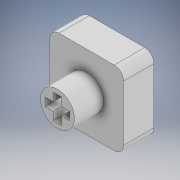
# Autodesk Inventor part: IPC STPT 4 key
Saved by Autodesk Inventor 2022 (Build 260153000, 153)
## iProperties
Created: 2021-12-31
Part Number: IPC STPT 4 key
Material: Generic
Document SubType Name: Modeling
Designer: solor
Density: 1 g/cm^3
Appearance: Default
Author: solor
Autodesk Inventor part; units mm, degrees
ref_plane "YZ Plane" through (0, 0, 0) normal (1, 0, 0) x (0, 1, 0)
ref_plane "XZ Plane" through (0, 0, 0) normal (0, 1, 0) x (-1, 0, 0)
sketch "Sketch1" plane through (0, 0, 0) normal (0, 0, 1) x (1, 0, 0)
  line L0 (14.6962, 12.74) -> (14.6962, 0) construction
  line L1 (10.61, 12.2) -> (1.53, 12.2)
  arc A0 (1.53, 12.2) -> (0, 10.67) centre (1.53, 10.67) ccw
  line L2 (0, 10.67) -> (0, 1.53)
  arc A1 (0, 1.53) -> (1.53, 0) centre (1.53, 1.53) ccw
  line L3 (1.53, 0) -> (10.61, 0)
  arc A2 (10.61, 0) -> (12.14, 1.53) centre (10.61, 1.53) ccw
  arc A3 (12.14, 10.67) -> (10.61, 12.2) centre (10.61, 10.67) ccw
  line L4 (12.14, 10.67) -> (12.14, 1.53)
  point P0 (0, 0)
  point P1 (0, 0)
  dimension "d10" = 12.74
  constraints: 10 end point, 8 point on circle, 4 centre point, 2 vertical, 1 point on line
  measures "d10" distance of L0.start L0.end
ref_plane "Work Plane1" through (0, 0, 5) normal (0, 0, 1) x (1, 0, 0)
sketch "Sketch2" plane through (0, 0, 5) normal (0, 0, 1) x (1, 0, 0)
  line L0 (10.88, 12.74) -> (1.8, 12.74) projected
  line L1 (10.88, 12.74) -> (1.8, 12.74) projected
  arc A0 (1.8, 12.74) -> (0, 10.94) centre (1.8, 10.94) ccw projected
  line L2 (0, 10.94) -> (0, 1.8) projected
  arc A1 (0, 1.8) -> (1.8, 0) centre (1.8, 1.8) ccw projected
  line L3 (1.8, 0) -> (10.88, 0) projected
  arc A2 (10.88, 0) -> (12.68, 1.8) centre (10.88, 1.8) ccw projected
  line L4 (12.68, 1.8) -> (12.68, 10.94) projected
  arc A3 (12.68, 10.94) -> (10.88, 12.74) centre (10.88, 10.94) ccw projected
  circle A4 centre (6.34, 6.37) radius 2.8
  line L5 (5.665, 8.395) -> (7.015, 8.395)
  line L6 (7.015, 4.345) -> (5.665, 4.345)
  line L7 (5.665, 4.345) -> (7.015, 8.395) construction
  line L8 (5.665, 8.395) -> (7.015, 4.345) construction
  line L9 (8.365, 5.695) -> (8.365, 7.045)
  line L10 (4.315, 7.045) -> (4.315, 5.695)
  line L11 (4.315, 5.695) -> (8.365, 7.045) construction
  line L12 (8.365, 5.695) -> (4.315, 7.045) construction
  line L13 (4.315, 5.695) -> (5.665, 5.695)
  line L14 (7.015, 5.695) -> (8.365, 5.695)
  line L15 (5.665, 4.345) -> (5.665, 5.695)
  line L16 (5.665, 7.045) -> (5.665, 8.395)
  line L17 (8.365, 7.045) -> (7.015, 7.045)
  line L18 (5.665, 7.045) -> (4.315, 7.045)
  line L19 (7.015, 8.395) -> (7.015, 7.045)
  line L20 (7.015, 5.695) -> (7.015, 4.345)
  point P0 (0, 0)
  dimension "d12" = 5
  dimension "d3" = 5.6
  dimension "d4" = 4.05
  dimension "d5" = 1.35
  dimension "d6" = 4.05
  dimension "d7" = 1.35
  constraints: 32 end point, 10 parallel, 8 perpendicular, 4 midpoint, 2 vertical, 1 centre point
  measures "d3" diameter of A4
  measures "d4" distance of L6.end L5.start
  measures "d5" distance of L5.start L5.end
  measures "d6" distance of L10.end L9.start
  measures "d7" distance of L9.end L9.start
extrude "Extrusion3" add sketch "Sketch1" along normal blind 5
sketch "Sketch3" plane through (0, 0, 5) normal (0, 0, 1) x (1, 0, 0)
  line L0 (10.61, 12.47) -> (1.53, 12.47)
  line L1 (10.61, 12.47) -> (1.53, 12.47)
  arc A0 (1.53, 12.47) -> (-0.27, 10.67) centre (1.53, 10.67) ccw
  line L2 (-0.27, 10.67) -> (-0.27, 1.53)
  arc A1 (-0.27, 1.53) -> (1.53, -0.27) centre (1.53, 1.53) ccw
  line L3 (1.53, -0.27) -> (10.61, -0.27)
  arc A2 (10.61, -0.27) -> (12.41, 1.53) centre (10.61, 1.53) ccw
  line L4 (12.41, 1.53) -> (12.41, 10.67)
  arc A3 (12.41, 10.67) -> (10.61, 12.47) centre (10.61, 10.67) ccw
  circle A4 centre (6.07, 6.1) radius 2.8
  line L5 (5.395, 8.125) -> (6.745, 8.125)
  line L6 (6.745, 4.075) -> (5.395, 4.075)
  line L7 (5.395, 4.075) -> (6.745, 8.125) construction
  line L8 (5.395, 8.125) -> (6.745, 4.075) construction
  line L9 (8.095, 5.425) -> (8.095, 6.775)
  line L10 (4.045, 6.775) -> (4.045, 5.425)
  line L11 (4.045, 5.425) -> (8.095, 6.775) construction
  line L12 (8.095, 5.425) -> (4.045, 6.775) construction
  line L13 (4.045, 5.425) -> (5.395, 5.425)
  line L14 (6.745, 5.425) -> (8.095, 5.425)
  line L15 (5.395, 4.075) -> (5.395, 5.425)
  line L16 (5.395, 6.775) -> (5.395, 8.125)
  line L17 (8.095, 6.775) -> (6.745, 6.775)
  line L18 (5.395, 6.775) -> (4.045, 6.775)
  line L19 (6.745, 8.125) -> (6.745, 6.775)
  line L20 (6.745, 5.425) -> (6.745, 4.075)
  line L21 (10.61, 12.2) -> (1.53, 12.2) projected
  line L22 (0, 10.67) -> (0, 1.53) projected
  point P0 (0, 0)
  point P1 (-0.27, -0.27)
  point P2 (6.07, 12.2)
  point P3 (0, 6.1)
  point P4 (6.07, 6.1)
  dimension "d14" = 5.6
  dimension "d15" = 4.05
  dimension "d16" = 1.35
  dimension "d17" = 4.05
  dimension "d18" = 1.35
  constraints: 42 end point, 10 parallel, 8 perpendicular, 8 point on circle, 6 midpoint, 5 centre point, 2 vertical
  measures "d14" diameter of A4
  measures "d15" distance of L6.end L5.start
  measures "d16" distance of L5.start L5.end
  measures "d17" distance of L10.end L9.start
  measures "d18" distance of L9.end L9.start
extrude "Extrusion4" add sketch "Sketch3" along normal blind 4.8 contours A4
sketch "Sketch4" plane through (0, 0, 0) normal (0, 0, -1) x (-1, 0, 0)
  line L0 (-13.9436, 0) -> (-13.9436, 2.266)
  line L1 (-15.5559, 0) -> (-15.5559, 6.84)
  line L2 (-1.53, 0) -> (-10.61, 0) projected
  line L3 (-11.3457, 9.9988) -> (-0.7943, 9.9988) construction
  line L4 (-0.7943, 9.9988) -> (-0.7943, 6.84) construction
  line L5 (-0.7943, 6.84) -> (-11.3457, 6.84) construction
  line L6 (-11.3457, 6.84) -> (-11.3457, 9.9988) construction
  line L7 (-7.4059, 5.3234) -> (-4.7341, 5.3234) construction
  line L8 (-4.7341, 5.3234) -> (-4.7341, 2.266) construction
  line L9 (-4.7341, 2.266) -> (-7.4059, 2.266) construction
  line L10 (-7.4059, 2.266) -> (-7.4059, 5.3234) construction
  spline S0 degree 2 poles (-10.0876, 6.84) (-10.4386, 6.84) (-10.9675, 6.9759) (-11.1949, 7.0748) knots 0 0 0 1 2 2 2
  line L11 (-11.1949, 7.0748) -> (-11.1949, 7.8015)
  line L12 (-11.1949, 7.8015) -> (-11.1257, 7.8015)
  spline S1 degree 2 poles (-11.1257, 7.8015) (-10.8959, 7.6062) (-10.3447, 7.3961) (-10.0852, 7.3961) knots 0 0 0 1 2 2 2
  spline S2 degree 2 poles (-10.0852, 7.3961) (-10.0184, 7.3961) (-9.8034, 7.4258) (-9.7391, 7.4554) knots 0 0 0 1 2 2 2
  spline S3 degree 2 poles (-9.7391, 7.4554) (-9.6601, 7.49) (-9.5488, 7.6161) (-9.5488, 7.7174) knots 0 0 0 1 2 2 2
  spline S4 degree 2 poles (-9.5488, 7.7174) (-9.5488, 7.8336) (-9.7293, 7.977) (-9.8528, 8.0091) knots 0 0 0 1 2 2 2
  spline S5 degree 2 poles (-9.8528, 8.0091) (-10.0086, 8.0511) (-10.362, 8.1228) (-10.5177, 8.1772) knots 0 0 0 1 2 2 2
  spline S6 degree 2 poles (-10.5177, 8.1772) (-10.8712, 8.3007) (-11.1776, 8.7234) (-11.1776, 9.0398) knots 0 0 0 1 2 2 2
  spline S7 degree 2 poles (-11.1776, 9.0398) (-11.1776, 9.4674) (-10.4534, 9.9988) (-9.9097, 9.9988) knots 0 0 0 1 2 2 2
  spline S8 degree 2 poles (-9.9097, 9.9988) (-9.6378, 9.9988) (-9.099, 9.8875) (-8.8864, 9.7936) knots 0 0 0 1 2 2 2
  line L13 (-8.8864, 9.7936) -> (-8.8864, 9.0966)
  line L14 (-8.8864, 9.0966) -> (-8.9532, 9.0966)
  spline S9 degree 2 poles (-8.9532, 9.0966) (-9.1237, 9.2424) (-9.6131, 9.4426) (-9.8701, 9.4426) knots 0 0 0 1 2 2 2
  spline S10 degree 2 poles (-9.8701, 9.4426) (-9.9715, 9.4426) (-10.1297, 9.413) (-10.2186, 9.3734) knots 0 0 0 1 2 2 2
  spline S11 degree 2 poles (-10.2186, 9.3734) (-10.2903, 9.3413) (-10.3941, 9.2128) (-10.3941, 9.1337) knots 0 0 0 1 2 2 2
  spline S12 degree 2 poles (-10.3941, 9.1337) (-10.3941, 9.015) (-10.2285, 8.8791) (-9.9913, 8.8247) knots 0 0 0 1 2 2 2
  spline S13 degree 2 poles (-9.9913, 8.8247) (-9.838, 8.7901) (-9.5538, 8.7234) (-9.3906, 8.6665) knots 0 0 0 1 2 2 2
  spline S14 degree 2 poles (-9.3906, 8.6665) (-9.0743, 8.5504) (-8.7653, 8.1648) (-8.7653, 7.8484) knots 0 0 0 1 2 2 2
  spline S15 degree 2 poles (-8.7653, 7.8484) (-8.7653, 7.3936) (-9.4796, 6.84) (-10.0876, 6.84) knots 0 0 0 1 2 2 2
  line L15 (-7.7866, 6.8944) -> (-7.7866, 9.3635)
  line L16 (-7.7866, 9.3635) -> (-8.6887, 9.3635)
  line L17 (-8.6887, 9.3635) -> (-8.6887, 9.9444)
  line L18 (-8.6887, 9.9444) -> (-6.1182, 9.9444)
  line L19 (-6.1182, 9.9444) -> (-6.1182, 9.3635)
  line L20 (-6.1182, 9.3635) -> (-7.0203, 9.3635)
  line L21 (-7.0203, 9.3635) -> (-7.0203, 6.8944)
  line L22 (-7.0203, 6.8944) -> (-7.7866, 6.8944)
  spline S16 degree 2 poles (-3.4587, 8.9829) (-3.4587, 8.7703) (-3.5947, 8.3848) (-3.7207, 8.2562) knots 0 0 0 1 2 2 2
  spline S17 degree 2 poles (-3.7207, 8.2562) (-3.7973, 8.1747) (-3.9852, 8.0412) (-4.0964, 7.9943) knots 0 0 0 1 2 2 2
  spline S18 degree 2 poles (-4.0964, 7.9943) (-4.2101, 7.9473) (-4.4746, 7.8929) (-4.6377, 7.8929) knots 0 0 0 1 2 2 2
  line L23 (-4.6377, 7.8929) -> (-5.0381, 7.8929)
  line L24 (-5.0381, 7.8929) -> (-5.0381, 6.8944)
  line L25 (-5.0381, 6.8944) -> (-5.8043, 6.8944)
  line L26 (-5.8043, 6.8944) -> (-5.8043, 9.9444)
  line L27 (-5.8043, 9.9444) -> (-4.6204, 9.9444)
  spline S19 degree 2 poles (-4.6204, 9.9444) (-4.3584, 9.9444) (-3.9753, 9.848) (-3.8196, 9.7442) knots 0 0 0 1 2 2 2
  spline S20 degree 2 poles (-3.8196, 9.7442) (-3.6466, 9.628) (-3.4587, 9.2474) (-3.4587, 8.9829) knots 0 0 0 1 2 2 2
  spline S21 degree 2 poles (-4.2447, 8.9631) (-4.2447, 9.0941) (-4.3683, 9.2795) (-4.4523, 9.3141) knots 0 0 0 1 2 2 2
  spline S22 degree 2 poles (-4.4523, 9.3141) (-4.5611, 9.3611) (-4.7588, 9.3759) (-4.9293, 9.3759) knots 0 0 0 1 2 2 2
  line L28 (-4.9293, 9.3759) -> (-5.0381, 9.3759)
  line L29 (-5.0381, 9.3759) -> (-5.0381, 8.4614)
  line L30 (-5.0381, 8.4614) -> (-4.9837, 8.4614)
  spline S23 degree 2 poles (-4.9837, 8.4614) (-4.8774, 8.4614) (-4.6846, 8.4663) (-4.613, 8.4787) knots 0 0 0 1 2 2 2
  spline S24 degree 2 poles (-4.613, 8.4787) (-4.5512, 8.4886) (-4.4152, 8.5479) (-4.3782, 8.585) knots 0 0 0 1 2 2 2
  spline S25 degree 2 poles (-4.3782, 8.585) (-4.2991, 8.6591) (-4.2447, 8.8247) (-4.2447, 8.9631) knots 0 0 0 1 2 2 2
  line L31 (-2.4626, 6.8944) -> (-2.4626, 9.3635)
  line L32 (-2.4626, 9.3635) -> (-3.3648, 9.3635)
  line L33 (-3.3648, 9.3635) -> (-3.3648, 9.9444)
  line L34 (-3.3648, 9.9444) -> (-0.7943, 9.9444)
  line L35 (-0.7943, 9.9444) -> (-0.7943, 9.3635)
  line L36 (-0.7943, 9.3635) -> (-1.6964, 9.3635)
  line L37 (-1.6964, 9.3635) -> (-1.6964, 6.8944)
  line L38 (-1.6964, 6.8944) -> (-2.4626, 6.8944)
  line L39 (-4.8181, 2.9852) -> (-5.2309, 2.9852)
  line L40 (-5.2309, 2.9852) -> (-5.2309, 2.266)
  line L41 (-5.2309, 2.266) -> (-5.9699, 2.266)
  line L42 (-5.9699, 2.266) -> (-5.9699, 2.9852)
  line L43 (-5.9699, 2.9852) -> (-7.3145, 2.9852)
  line L44 (-7.3145, 2.9852) -> (-7.3145, 3.5537)
  line L45 (-7.3145, 3.5537) -> (-5.9946, 5.3234)
  line L46 (-5.9946, 5.3234) -> (-5.2309, 5.3234)
  line L47 (-5.2309, 5.3234) -> (-5.2309, 3.5339)
  line L48 (-5.2309, 3.5339) -> (-4.8181, 3.5339)
  line L49 (-4.8181, 3.5339) -> (-4.8181, 2.9852)
  line L50 (-5.9699, 3.5339) -> (-5.9699, 4.572)
  line L51 (-5.9699, 4.572) -> (-6.7435, 3.5339)
  line L52 (-6.7435, 3.5339) -> (-5.9699, 3.5339)
  point P0 (0, 0)
  point P1 (-6.07, 0)
  point P2 (-6.07, 2.266)
  point P3 (-6.07, 6.84)
  point P4 (-6.07, 6.84)
  point P5 (-6.07, 2.266)
  dimension "d21" = 2.266
  dimension "d22" = 6.84
  constraints: 4 end point, 3 midpoint, 2 vertical, 4 other
  measures "d21" distance of L0.start L0.end
  measures "d22" distance of L1.start L1.end
sketch "Sketch5" plane through (0, 0, 0) normal (0, 0, -1) x (-1, 0, 0)
  point P0 (0, 0)
extrude "Extrusion5" add sketch "Sketch4" along normal blind 0.9
body "Solid2"
